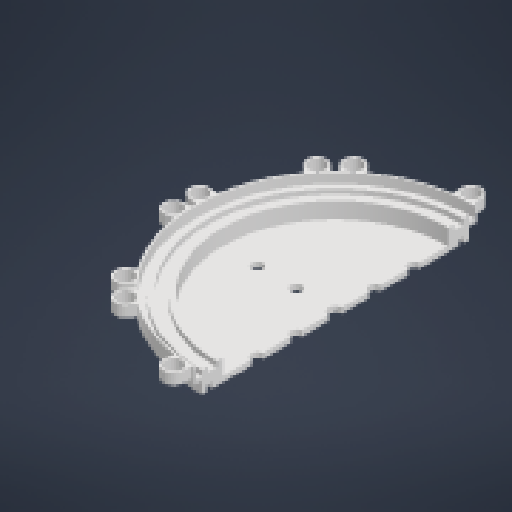
# Autodesk Inventor part: base frame
Saved by Autodesk Inventor 2026 (Build 300175050, 175E)
## iProperties
Created: 2026-03-26
Part Number: base frame
Material: Generic
Document SubType Name: Modeling
Designer: sniel
Density: 1 g/cm^3
Appearance: Default
Author: sniel
Autodesk Inventor part; units mm, degrees
ref_plane "YZ Plane" through (0, 0, 0) normal (1, 0, 0) x (0, 1, 0)
ref_plane "XZ Plane" through (0, 0, 0) normal (0, 1, 0) x (-1, 0, 0)
ref_plane "XY Plane" through (0, 0, 0) normal (0, 0, 1) x (1, 0, 0)
sketch "Sketch1" plane through (0, 0, 0) normal (0, 0, 1) x (1, 0, 0)
  line L0 (-117.014, 29.8572) -> (-117.014, 27.8572)
  line L1 (-119.014, 27.8572) -> (-119.014, 29.8572)
  line L2 (-0.014, 29.8572) -> (-125.014, 29.8572)
  line L3 (-0.014, 27.8572) -> (-119.014, 27.8572)
  line L4 (-113.014, 27.8572) -> (-113.014, 29.8572)
  line L5 (-111.014, 29.8572) -> (-111.014, 27.8572)
  line L6 (-105.014, 14.8572) -> (-105.014, 29.8572)
  line L7 (-0.014, 34.8572) -> (-130.014, 34.8572)
  line L8 (-100.014, 34.8572) -> (-100.014, 19.8572)
  line L9 (-130.014, 24.8572) -> (-130.014, 34.8572)
  line L10 (-0.014, 24.8572) -> (-130.014, 24.8572)
  line L11 (-0.014, 14.8572) -> (-105.014, 14.8572)
  line L12 (-100.014, 19.8572) -> (-0.014, 19.8572)
  line L13 (-125.014, 29.8572) -> (-125.014, 24.8572)
  line L14 (-125.014, 29.8572) -> (-124.814, 29.8572)
  line L15 (-124.814, 29.8572) -> (-124.814, 29.6572)
  line L16 (-124.814, 29.6572) -> (-125.014, 29.6572)
  line L17 (-125.014, 29.6572) -> (-125.014, 29.8572)
  line L18 (-119.014, 29.8572) -> (-119.214, 29.8572)
  line L19 (-119.214, 29.8572) -> (-119.214, 29.6572)
  line L20 (-119.214, 29.6572) -> (-119.014, 29.6572)
  line L21 (-119.014, 29.6572) -> (-119.014, 29.8572)
  line L22 (-111.014, 29.8572) -> (-110.814, 29.8572)
  line L23 (-110.814, 29.8572) -> (-110.814, 29.6572)
  line L24 (-110.814, 29.6572) -> (-111.014, 29.6572)
  line L25 (-111.014, 29.6572) -> (-111.014, 29.8572)
  line L26 (-105.014, 29.8572) -> (-105.214, 29.8572)
  line L27 (-105.214, 29.8572) -> (-105.214, 29.6572)
  line L28 (-105.214, 29.6572) -> (-105.014, 29.6572)
  line L29 (-105.014, 29.6572) -> (-105.014, 29.8572)
  line L30 (-124.814, 29.6572) -> (-119.214, 29.6572)
  line L31 (-119.214, 29.6572) -> (-119.214, 9.6572)
  line L32 (-119.214, 9.6572) -> (-124.814, 9.6572)
  line L33 (-124.814, 9.6572) -> (-124.814, 29.6572)
  line L34 (-110.814, 29.6572) -> (-105.214, 29.6572)
  line L35 (-105.214, 29.6572) -> (-105.214, 9.6572)
  line L36 (-105.214, 9.6572) -> (-110.814, 9.6572)
  line L37 (-110.814, 9.6572) -> (-110.814, 29.6572)
  line L38 (-119.014, 27.8572) -> (-117.014, 27.8572)
  line L39 (-117.014, 27.8572) -> (-117.014, 26.8572)
  line L40 (-117.014, 26.8572) -> (-119.014, 26.8572)
  line L41 (-119.014, 26.8572) -> (-119.014, 27.8572)
  line L42 (-113.014, 27.8572) -> (-111.014, 27.8572)
  line L43 (-111.014, 27.8572) -> (-111.014, 26.8572)
  line L44 (-111.014, 26.8572) -> (-113.014, 26.8572)
  line L45 (-113.014, 26.8572) -> (-113.014, 27.8572)
  line L46 (-119.214, 26.8572) -> (-110.814, 26.8572)
  line L47 (-110.814, 26.8572) -> (-110.814, 24.8572)
  line L48 (-110.814, 24.8572) -> (-119.214, 24.8572)
  line L49 (-119.214, 24.8572) -> (-119.214, 26.8572)
  line L50 (-124.814, 9.6572) -> (-0.014, 9.6572)
  line L51 (-0.014, 9.6572) -> (-0.014, 14.6572)
  line L52 (-0.014, 14.6572) -> (-124.814, 14.6572)
  line L53 (-124.814, 14.6572) -> (-124.814, 9.6572)
  line L54 (-124.814, 24.8572) -> (-125.014, 24.8572)
  line L55 (-125.014, 24.8572) -> (-125.014, 24.6572)
  line L56 (-125.014, 24.6572) -> (-124.814, 24.6572)
  line L57 (-124.814, 24.6572) -> (-124.814, 24.8572)
  line L58 (-124.814, 24.6572) -> (-132.014, 24.6572)
  line L59 (-132.014, 24.6572) -> (-132.014, 20.6572)
  line L60 (-132.014, 20.6572) -> (-124.814, 20.6572)
  line L61 (-124.814, 20.6572) -> (-124.814, 24.6572)
  line L62 (-132.014, 24.6572) -> (-130.214, 24.6572)
  line L63 (-130.214, 24.6572) -> (-130.214, 34.8572)
  line L64 (-130.214, 34.8572) -> (-132.014, 34.8572)
  line L65 (-132.014, 34.8572) -> (-132.014, 24.6572)
  line L66 (-0.014, 9.6572) -> (-6.014, 9.6572)
  line L67 (-6.014, 9.6572) -> (-6.014, 14.6572)
  line L68 (-6.014, 14.6572) -> (-0.014, 14.6572)
  line L69 (-0.014, 14.6572) -> (-0.014, 9.6572)
  line L70 (-119.014, 27.3572) -> (-117.014, 27.3572)
  line L71 (-117.014, 27.3572) -> (-117.014, 26.8572)
  line L72 (-117.014, 26.8572) -> (-119.014, 26.8572)
  line L73 (-119.014, 26.8572) -> (-119.014, 27.3572)
  line L74 (-113.014, 27.3572) -> (-111.014, 27.3572)
  line L75 (-111.014, 27.3572) -> (-111.014, 26.8572)
  line L76 (-111.014, 26.8572) -> (-113.014, 26.8572)
  line L77 (-113.014, 26.8572) -> (-113.014, 27.3572)
  line L78 (0, -6.9714) -> (0, 41.8287) projected
  line L79 (-115.014, 29.8572) -> (-115.014, 24.3572)
  line L80 (-110.814, 23.8572) -> (-119.214, 23.8572)
  line L81 (-110.814, 26.8572) -> (-113.014, 26.8572)
  line L82 (-113.014, 26.8572) -> (-113.014, 23.8572)
  line L83 (-113.014, 23.8572) -> (-110.814, 23.8572)
  line L84 (-110.814, 23.8572) -> (-110.814, 26.8572)
  line L85 (-117.014, 26.8572) -> (-119.214, 26.8572)
  line L86 (-119.214, 26.8572) -> (-119.214, 23.8572)
  line L87 (-119.214, 23.8572) -> (-117.014, 23.8572)
  line L88 (-117.014, 23.8572) -> (-117.014, 26.8572)
  line L89 (-110.814, 24.3572) -> (-119.214, 24.3572)
  point P0 (0, 0)
  point P1 (-105.214, 14.6572)
  point P2 (-113.014, 24.8572)
  point P3 (-115.014, 23.8572)
  point P4 (-115.014, 24.8572)
  point P5 (-117.014, 24.8572)
  dimension "d0" = 0.2
  dimension "d1" = 0.2
  dimension "d2" = 0.2
  dimension "d3" = 0.2
  dimension "d4" = 0.2
  dimension "d5" = 0.2
  dimension "d6" = 0.2
  dimension "d7" = 0.2
  dimension "d8" = 20
  dimension "d9" = 20
  dimension "d10" = 1
  dimension "d11" = 1
  dimension "d12" = 2
  dimension "d13" = 5
  dimension "d14" = 0.2
  dimension "d15" = 7.2
  dimension "d16" = 4
  dimension "d17" = 1.8
  dimension "d18" = 6
  dimension "d86" = 5.5
  constraints: 178 end point, 36 parallel, 20 perpendicular, 18 horizontal, 11 point on line, 2 midpoint, 1 vertical
  measures "d0" distance of L15.end L16.end
  measures "d1" distance of L14.end L15.end
  measures "d2" distance of L20.end L19.end
  measures "d3" distance of L19.end L18.end
  measures "d4" distance of L23.end L24.end
  measures "d5" distance of L22.end L23.end
  measures "d6" distance of L28.end L27.end
  measures "d7" distance of L27.end L26.end
  measures "d8" distance of L30.end L31.end
  measures "d9" distance of L34.end L35.end
  measures "d10" distance of L38.end L39.end
  measures "d11" distance of L42.end L43.end
  measures "d12" distance of L46.end L47.end
  measures "d13" distance of L51.end L50.end
  measures "d14" distance of L55.end L54.end
  measures "d15" distance of L60.end L59.end
  measures "d16" distance of L59.end L58.end
  measures "d17" distance of L64.end L63.end
  measures "d18" distance of L67.end L68.end
  measures "d86" distance of L79.start L79.end
revolve "Revolution1" add sketch "Sketch1" angle 360 about axis through (0, -10, 0) along (0, 1, 0) contours L31 L10 L33 L30 | L79 L89 L88 L10 | L10 L82 L89 L79 | L88 L89 L31 L10 | L37 L34 L35 L3 | L3 L35 L10 L37 | L10 L37 L89 L82 | L89 L82 L80 L88 | L31 L52 L33 L10 | L88 L80 L31 L89 | L10 L35 L52 L37 | L89 L37 L80 L82 | L80 L37 L52 L31 | L33 L60 L59 L58 L56 | L52 L67 L50 L35 | L35 L36 L37 L52 | L52 L37 L50 L31 | L31 L32 L33 L52 | L58 L65 L64 L63
sketch "Sketch3" plane through (0, 29.6572, 0) normal (0, 1, 0) x (1, 0, 0)
  circle A0 centre (0, 0) radius 132.014 projected
  circle A1 centre (0, 0) radius 6.014 projected
  line L0 (0, 0) -> (-93.348, -93.348)
  line L1 (0, 0) -> (132.014, 0) construction
  line L2 (0, 0) -> (0, -132.014)
  line L3 (0, 0) -> (-84.857, -101.1286)
  line L4 (0, 0) -> (160.5313, 0) construction
  line L5 (-84.857, -101.1286) -> (-94.4988, -112.6193)
  circle A2 centre (0, 0) radius 130.214 projected
  line L6 (0, 0) -> (-11.5058, -131.5116)
  line L7 (0, 0) -> (132.014, 0) construction
  line L8 (-11.5058, -131.5116) -> (-12.8131, -146.4546)
  circle A3 centre (-12.1594, -138.9831) radius 7.5
  circle A4 centre (-89.6779, -106.8739) radius 7.5
  circle A5 centre (-12.1594, -138.9831) radius 9.3
  circle A6 centre (-89.6779, -106.8739) radius 9.3
  circle A7 centre (0, 0) radius 139.514
  line L9 (-2.873, -139.4844) -> (0, 0)
  line L10 (-21.3919, -137.8642) -> (0, 0)
  line L11 (-82.3584, -112.6111) -> (0, 0)
  line L12 (-96.5989, -100.6619) -> (0, 0)
  point P0 (-91.4059, -95.2505)
  point P1 (-77.9309, -106.5573)
  point P2 (-2.7185, -131.986)
  point P3 (-20.2419, -130.4529)
  dimension "d22" = 135
  dimension "d23" = 130
  dimension "d24" = 15
  dimension "d25" = 95
  dimension "d26" = 15
  constraints: 26 end point, 13 point on circle, 3 centre point, 3 coincident, 3 horizontal, 2 equal length, 2 midpoint, 1 vertical, 6 other
  measures "d22" angle of L0 L1
  measures "d23" angle of L3 L4
  measures "d24" distance of L3.end L5.end
  measures "d25" angle of L6 L7
  measures "d26" distance of L6.end L8.end
extrude "Extrusion2" add sketch "Sketch3" along normal mid plane 10.4 contours A0 A6 L12 | L9 A5 A0 | A0 A4 A7 L12 A6 | A5 L9 A7 A3 A0 | A6 A0 L11 | A0 A6 A7 A4 | A7 A4 A6 | A3 A7 A5 A0 | A5 A7 A3 | A5 L10 A0
pattern_circular "Circular Pattern1" count 8 over 360 about axis through (0, -10, 0) along (0, 1, 0) of "Extrusion2"
sketch "Sketch5" plane through (0, 9.6572, 0) normal (0, -1, 0) x (1, 0, 0)
  circle A0 centre (0, 0) radius 132.014 projected
  arc A1 (-2.7185, -131.986) -> (2.7185, -131.986) centre (0, 0) ccw projected
  line L0 (0, -10) -> (26.9875, -10) construction
  line L1 (41.275, 0) -> (-30.9983, 0)
  line L2 (-7.5, -120.025) -> (7.5, -120.025)
  line L3 (7.5, -120.025) -> (7.5, -115.025)
  line L4 (7.5, -115.025) -> (-7.5, -115.025)
  line L5 (-7.5, -115.025) -> (-7.5, -120.025)
  line L6 (-7.5, -120.025) -> (7.5, -115.025) construction
  line L7 (7.5, -120.025) -> (-7.5, -115.025) construction
  line L8 (10, -122.525) -> (5, -122.525)
  line L9 (5, -122.525) -> (5, -112.525)
  line L10 (5, -112.525) -> (10, -112.525)
  line L11 (10, -112.525) -> (10, -122.525)
  line L12 (10, -122.525) -> (5, -112.525) construction
  line L13 (5, -122.525) -> (10, -112.525) construction
  line L14 (-5, -122.525) -> (-10, -122.525)
  line L15 (-10, -122.525) -> (-10, -112.525)
  line L16 (-10, -112.525) -> (-5, -112.525)
  line L17 (-5, -112.525) -> (-5, -122.525)
  line L18 (-5, -122.525) -> (-10, -112.525) construction
  line L19 (-10, -122.525) -> (-5, -112.525) construction
  line L20 (0, 0) -> (0, -115)
  line L21 (5, 112.525) -> (10, 112.525)
  line L22 (-10, 122.525) -> (-10, 112.525)
  line L23 (7.5, 115.025) -> (-7.5, 115.025)
  line L24 (-7.5, 115.025) -> (-7.5, 120.025)
  line L25 (-7.5, 120.025) -> (7.5, 120.025)
  line L26 (7.5, 120.025) -> (7.5, 115.025)
  line L27 (-7.5, 120.025) -> (7.5, 115.025) construction
  line L28 (7.5, 120.025) -> (-7.5, 115.025) construction
  line L29 (10, 122.525) -> (5, 122.525)
  line L30 (10, 112.525) -> (10, 122.525)
  line L31 (10, 122.525) -> (5, 112.525) construction
  line L32 (5, 122.525) -> (10, 112.525) construction
  line L33 (5, 122.525) -> (5, 112.525)
  line L34 (-5, 122.525) -> (-10, 122.525)
  line L35 (-5, 112.525) -> (-5, 122.525)
  line L36 (-5, 122.525) -> (-10, 112.525) construction
  line L37 (-10, 122.525) -> (-5, 112.525) construction
  line L38 (-10, 112.525) -> (-5, 112.525)
  line L39 (0, 0) -> (0, 115)
  arc A2 (131.986, -2.7185) -> (131.986, 2.7185) centre (0, 0) ccw
  line L40 (10, 0) -> (10, 26.9875) construction
  line L41 (0, 41.275) -> (0, -30.9983)
  line L42 (112.525, 5) -> (112.525, 10)
  line L43 (122.525, -10) -> (112.525, -10)
  line L44 (115.025, 7.5) -> (115.025, -7.5)
  line L45 (115.025, -7.5) -> (120.025, -7.5)
  line L46 (120.025, -7.5) -> (120.025, 7.5)
  line L47 (120.025, 7.5) -> (115.025, 7.5)
  line L48 (120.025, -7.5) -> (115.025, 7.5) construction
  line L49 (120.025, 7.5) -> (115.025, -7.5) construction
  line L50 (122.525, 10) -> (122.525, 5)
  line L51 (112.525, 10) -> (122.525, 10)
  line L52 (122.525, 10) -> (112.525, 5) construction
  line L53 (122.525, 5) -> (112.525, 10) construction
  line L54 (122.525, 5) -> (112.525, 5)
  line L55 (122.525, -5) -> (122.525, -10)
  line L56 (112.525, -5) -> (122.525, -5)
  line L57 (122.525, -5) -> (112.525, -10) construction
  line L58 (122.525, -10) -> (112.525, -5) construction
  line L59 (112.525, -10) -> (112.525, -5)
  line L60 (0, 0) -> (115, 0)
  line L61 (-122.525, 5) -> (-112.525, 5)
  line L62 (-120.025, 7.5) -> (-115.025, 7.5)
  line L63 (-120.025, -7.5) -> (-115.025, 7.5) construction
  line L64 (-120.025, 7.5) -> (-115.025, -7.5) construction
  line L65 (-112.525, 5) -> (-112.525, 10)
  line L66 (-112.525, 10) -> (-122.525, 10)
  line L67 (-122.525, 10) -> (-112.525, 5) construction
  line L68 (-122.525, 5) -> (-112.525, 10) construction
  line L69 (-120.025, -7.5) -> (-120.025, 7.5)
  line L70 (-122.525, 10) -> (-122.525, 5)
  line L71 (0, 0) -> (-115, 0)
  line L72 (-115.025, 7.5) -> (-115.025, -7.5)
  line L73 (-115.025, -7.5) -> (-120.025, -7.5)
  line L74 (-112.525, -5) -> (-122.525, -5)
  line L75 (-122.525, -5) -> (-122.525, -10)
  line L76 (-122.525, -10) -> (-112.525, -5) construction
  line L77 (-112.525, -10) -> (-112.525, -5)
  line L78 (-122.525, -5) -> (-112.525, -10) construction
  line L79 (-122.525, -10) -> (-112.525, -10)
  point P0 (7.5, -117.525)
  point P1 (-7.5, -117.525)
  point P2 (-5, -120.025)
  point P3 (5, -120.025)
  point P4 (5, -115.025)
  point P5 (-5, -115.025)
  point P6 (-7.5, 117.525)
  point P7 (7.5, 117.525)
  point P8 (-5, 115.025)
  point P9 (5, 115.025)
  point P10 (5, 120.025)
  point P11 (-5, 120.025)
  point P12 (0, 0)
  point P13 (0, 0)
  point P14 (117.525, -7.5)
  point P15 (117.525, 7.5)
  point P16 (-117.525, 7.5)
  point P17 (-117.525, -7.5)
  point P18 (120.025, -5)
  point P19 (120.025, 5)
  point P20 (115.025, 5)
  point P21 (115.025, -5)
  point P22 (-120.025, 5)
  point P23 (-120.025, -5)
  point P24 (-115.025, -5)
  point P25 (-115.025, 5)
  dimension "d62" = 115
  dimension "d89" = 115
  constraints: 160 end point, 30 symmetric about line, 2 horizontal, 2 perpendicular, 2 point on circle, 1 centre point
  measures "d62" distance of L20.start L20.end
  measures "d89" distance of L60.start L60.end
extrude "Extrusion4" cut sketch "Sketch5" against normal blind 5 contours L5 L4 L17 L2 | L2 L17 L14 L15 L16 L4 L5 | L17 L4 L9 L2 | L9 L4 L3 L2 | L2 L3 L4 L9 L10 L11 L8 | L33 L23 L26 L25 L29 L30 L21 | L33 L25 L26 L23 | L23 L35 L25 L33 | L35 L38 L22 L34 L25 L24 L23 | L23 L24 L25 L35 | L42 L51 L50 L54 L46 L47 L44 | L54 L46 L56 L44 | L44 L47 L46 L54 | L56 L46 L45 L44 | L44 L45 L46 L56 L55 L43 L59 | L70 L66 L65 L61 L72 L62 L69 | L69 L62 L72 L61 | L61 L72 L74 L69 | L74 L72 L73 L69 | L69 L73 L72 L74 L77 L79 L75
sketch "Sketch6" plane through (0, 9.6572, 0) normal (0, -1, 0) x (1, 0, 0)
  arc A0 (-5.3566, 19.1544) -> (-6.464, 18.848) centre (-0.6442, -0.0297) ccw projected
  arc A1 (-3.9705, 16.9967) -> (-5.3566, 19.1544) centre (-15.5742, 11.0669) ccw projected
  arc A2 (-3.9236, 16.861) -> (-3.9705, 16.9967) centre (-22.8251, 10.402) ccw projected
  arc A3 (-3.9028, 16.8624) -> (-3.9236, 16.861) centre (2.0614, -72.6393) ccw projected
  arc A4 (-3.6762, 16.3816) -> (-3.9028, 16.8624) centre (-15.5742, 11.0669) ccw projected
  arc A5 (-2.7169, 16.5302) -> (-3.6762, 16.3816) centre (-0.6442, -0.0297) ccw projected
  arc A6 (-1.9537, 19.6813) -> (-2.7169, 16.5302) centre (10.2313, 15.0621) ccw projected
  arc A7 (-0.8054, 19.724) -> (-1.9537, 19.6813) centre (-0.6442, -0.0297) ccw projected
  arc A8 (0.1902, 16.6385) -> (-0.8054, 19.724) centre (-12.6127, 14.2109) ccw projected
  arc A9 (1.158, 16.5618) -> (0.1902, 16.6385) centre (-0.6442, -0.0297) ccw projected
  arc A10 (1.3482, 17.0581) -> (1.158, 16.5618) centre (13.4185, 12.1472) ccw projected
  arc A11 (1.369, 17.0582) -> (1.3482, 17.0581) centre (2.0614, -72.6393) ccw projected
  arc A12 (1.4057, 17.197) -> (1.369, 17.0582) centre (20.6987, 12.0238) ccw projected
  arc A13 (2.6273, 19.4519) -> (1.4057, 17.197) centre (13.4185, 12.1472) ccw projected
  arc A14 (3.7545, 19.2287) -> (2.6273, 19.4519) centre (-0.6442, -0.0297) ccw projected
  arc A15 (4.0117, 15.9968) -> (3.7545, 19.2287) centre (-9.006, 16.5872) ccw projected
  arc A16 (4.9357, 15.6989) -> (4.0117, 15.9968) centre (-0.6442, -0.0297) ccw projected
  arc A17 (7.0319, 18.1723) -> (4.9357, 15.6989) centre (15.8477, 8.5759) ccw projected
  arc A18 (8.0773, 17.6952) -> (7.0319, 18.1723) centre (-0.6442, -0.0297) ccw projected
  arc A19 (7.5821, 14.491) -> (8.0773, 17.6952) centre (-4.9485, 18.0676) ccw projected
  arc A20 (8.4125, 13.9881) -> (7.5821, 14.491) centre (-0.6442, -0.0297) ccw projected
  arc A21 (11.0227, 15.9114) -> (8.4125, 13.9881) centre (17.3877, 4.5407) ccw projected
  arc A22 (11.9298, 15.2061) -> (11.0227, 15.9114) centre (-0.6442, -0.0297) ccw projected
  arc A23 (10.7091, 12.2025) -> (11.9298, 15.2061) centre (-0.6589, 18.5724) ccw projected
  arc A24 (11.4012, 11.5216) -> (10.7091, 12.2025) centre (-0.6442, -0.0297) ccw projected
  arc A25 (14.3845, 12.7912) -> (11.4012, 11.5216) centre (17.9557, 0.259) ccw projected
  arc A26 (15.1045, 11.8956) -> (14.3845, 12.7912) centre (-0.6442, -0.0297) ccw projected
  arc A27 (13.224, 9.2545) -> (15.1045, 11.8956) centre (3.6314, 18.0744) ccw projected
  arc A28 (13.7404, 8.4324) -> (13.224, 9.2545) centre (-0.6442, -0.0297) ccw projected
  arc A29 (16.9361, 8.9797) -> (13.7404, 8.4324) centre (17.5209, -4.0382) ccw projected
  arc A30 (17.4302, 7.9423) -> (16.9361, 8.9797) centre (-0.6442, -0.0297) ccw projected
  arc A31 (14.9913, 5.806) -> (17.4302, 7.9423) centre (7.6912, 16.6004) ccw projected
  arc A32 (15.3042, 4.887) -> (14.9913, 5.806) centre (-0.6442, -0.0297) ccw projected
  arc A33 (18.5399, 4.6826) -> (15.3042, 4.887) centre (16.1068, -8.1193) ccw projected
  arc A34 (18.7815, 3.5591) -> (18.5399, 4.6826) centre (-0.6442, -0.0297) ccw projected
  arc A35 (15.9157, 2.0429) -> (18.7815, 3.5591) centre (11.3017, 14.2298) ccw projected
  arc A36 (16.0081, 1.0765) -> (15.9157, 2.0429) centre (-0.6442, -0.0297) ccw projected
  arc A37 (19.1095, 0.1314) -> (16.0081, 1.0765) centre (13.7897, -11.7644) ccw projected
  arc A38 (19.0855, -1.0175) -> (19.1095, 0.1314) centre (-0.6442, -0.0297) ccw projected
  arc A39 (15.9473, -1.832) -> (19.0855, -1.0175) centre (14.2682, 11.0905) ccw projected
  arc A40 (15.8144, -2.7936) -> (15.9473, -1.832) centre (-0.6442, -0.0297) ccw projected
  arc A41 (18.6142, -4.4285) -> (15.8144, -2.7936) centre (10.6945, -14.7767) ccw projected
  arc A42 (18.3259, -5.5408) -> (18.6142, -4.4285) centre (-0.6442, -0.0297) ccw projected
  arc A43 (15.0844, -5.6096) -> (18.3259, -5.5408) centre (16.4307, 7.3517) ccw projected
  arc A44 (14.7334, -6.5147) -> (15.0844, -5.6096) centre (-0.6442, -0.0297) ccw projected
  arc A45 (17.0807, -8.7512) -> (14.7334, -6.5147) centre (6.9879, -16.9941) ccw projected
  arc A46 (16.5436, -9.7671) -> (17.0807, -8.7512) centre (-0.6442, -0.0297) ccw projected
  arc A47 (13.3736, -9.0865) -> (16.5436, -9.7671) centre (17.6728, 3.215) ccw projected
  arc A48 (12.8233, -9.8863) -> (13.3736, -9.0865) centre (-0.6442, -0.0297) ccw projected
  arc A49 (14.5916, -12.6038) -> (12.8233, -9.8863) centre (2.8699, -18.2969) ccw projected
  arc A50 (13.8347, -13.4684) -> (14.5916, -12.6038) centre (-0.6442, -0.0297) ccw projected
  arc A51 (10.9071, -12.0751) -> (13.8347, -13.4684) centre (17.9273, -1.0967) ccw projected
  arc A52 (10.1872, -12.7264) -> (10.9071, -12.0751) centre (-0.6442, -0.0297) ccw projected
  arc A53 (11.2811, -15.7785) -> (10.1872, -12.7264) centre (-1.4375, -18.615) ccw projected
  arc A54 (10.3453, -16.4452) -> (11.2811, -15.7785) centre (-0.6442, -0.0297) ccw projected
  arc A55 (7.8179, -14.4144) -> (10.3453, -16.4452) centre (17.1806, -5.3508) ccw projected
  arc A56 (6.9672, -14.8821) -> (7.8179, -14.4144) centre (-0.6442, -0.0297) ccw projected
  arc A57 (7.3278, -18.1042) -> (6.9672, -14.8821) centre (-5.7022, -17.9311) ccw projected
  arc A58 (6.2634, -18.5371) -> (7.3278, -18.1042) centre (-0.6442, -0.0297) ccw projected
  arc A59 (4.2725, -15.9781) -> (6.2634, -18.5371) centre (15.4731, -9.3181) ccw projected
  arc A60 (3.3369, -16.237) -> (4.2725, -15.9781) centre (-0.6442, -0.0297) ccw projected
  arc A61 (2.9446, -19.4554) -> (3.3369, -16.237) centre (-9.6942, -16.2821) ccw projected
  arc A62 (1.8091, -19.6312) -> (2.9446, -19.4554) centre (-0.6442, -0.0297) ccw projected
  arc A63 (0.462, -16.6821) -> (1.8091, -19.6312) centre (12.8966, -12.7846) ccw projected
  arc A64 (-0.5081, -16.7183) -> (0.462, -16.6821) centre (-0.6442, -0.0297) ccw projected
  arc A65 (-1.632, -19.7595) -> (-0.5081, -16.7183) centre (-13.1983, -13.757) ccw projected
  arc A66 (-2.7775, -19.6687) -> (-1.632, -19.7595) centre (-0.6442, -0.0297) ccw projected
  arc A67 (-3.4081, -16.4884) -> (-2.7775, -19.6687) centre (9.5901, -15.5635) ccw projected
  arc A68 (-4.3604, -16.2998) -> (-3.4081, -16.4884) centre (-0.6442, -0.0297) ccw projected
  arc A69 (-6.1553, -18.9999) -> (-4.3604, -16.2998) centre (-16.0256, -10.4918) ccw projected
  arc A70 (-7.249, -18.6473) -> (-6.1553, -18.9999) centre (-0.6442, -0.0297) ccw projected
  arc A71 (-7.1292, -15.4073) -> (-7.249, -18.6473) centre (5.7319, -17.505) ccw projected
  arc A72 (-8.0124, -15.0042) -> (-7.1292, -15.4073) centre (-0.6442, -0.0297) ccw projected
  arc A73 (-10.3816, -17.2176) -> (-8.0124, -15.0042) centre (-18.0237, -6.6626) ccw projected
  arc A74 (-11.3645, -16.6223) -> (-10.3816, -17.2176) centre (-0.6442, -0.0297) ccw projected
  arc A75 (-10.5008, -13.4973) -> (-11.3645, -16.6223) centre (1.5299, -18.5044) ccw projected
  arc A76 (-11.2672, -12.9014) -> (-10.5008, -13.4973) centre (-0.6442, -0.0297) ccw projected
  arc A77 (-14.0829, -14.5087) -> (-11.2672, -12.9014) centre (-19.0849, -2.4758) ccw projected
  arc A78 (-14.9021, -13.7028) -> (-14.0829, -14.5087) centre (-0.6442, -0.0297) ccw projected
  arc A79 (-13.3409, -10.8612) -> (-14.9021, -13.7028) centre (-2.7892, -18.5078) ccw projected
  arc A80 (-13.9492, -10.1046) -> (-13.3409, -10.8612) centre (-0.6442, -0.0297) ccw projected
  arc A81 (-17.0597, -11.0192) -> (-13.9492, -10.1046) centre (-19.1519, 1.8428) ccw projected
  arc A82 (-17.671, -10.0462) -> (-17.0597, -11.0192) centre (-0.6442, -0.0297) ccw projected
  arc A83 (-15.4966, -7.6412) -> (-17.671, -10.0462) centre (-6.9927, -17.5151) ccw projected
  arc A84 (-15.914, -6.7647) -> (-15.4966, -7.6412) centre (-0.6442, -0.0297) ccw projected
  arc A85 (-19.1516, -6.9373) -> (-15.914, -6.7647) centre (-18.2212, 6.0605) ccw projected
  arc A86 (-19.5219, -5.8495) -> (-19.1516, -6.9373) centre (-0.6442, -0.0297) ccw projected
  arc A87 (-16.8515, -4.0108) -> (-19.5219, -5.8495) centre (-10.854, -15.5797) ccw projected
  arc A88 (-17.0556, -3.0617) -> (-16.8515, -4.0108) centre (-0.6442, -0.0297) ccw projected
  arc A89 (-20.2457, -2.483) -> (-17.0556, -3.0617) centre (-16.3429, 9.9499) ccw projected
  arc A90 (-20.3552, -1.3392) -> (-20.2457, -2.483) centre (-0.6442, -0.0297) ccw projected
  arc A91 (-17.3328, -0.1659) -> (-20.3552, -1.3392) centre (-14.1649, -12.806) ccw projected
  arc A92 (-17.3125, 0.8047) -> (-17.3328, -0.1659) centre (-0.6442, -0.0297) ccw projected
  arc A93 (-20.2832, 2.1035) -> (-17.3125, 0.8047) centre (-13.6183, 13.3012) ccw projected
  arc A94 (-20.1259, 3.2418) -> (-20.2832, 2.1035) centre (-0.6442, -0.0297) ccw projected
  arc A95 (-16.9143, 3.6865) -> (-20.1259, 3.2418) centre (-16.7468, -9.3435) ccw projected
  arc A96 (-16.6707, 4.6262) -> (-16.9143, 3.6865) centre (-0.6442, -0.0297) ccw projected
  arc A97 (-19.2618, 6.5751) -> (-16.6707, 4.6262) centre (-10.1942, 15.9339) ccw projected
  arc A98 (-18.8463, 7.6464) -> (-19.2618, 6.5751) centre (-0.6442, -0.0297) ccw projected
  arc A99 (-15.6188, 7.3384) -> (-18.8463, 7.6464) centre (-18.4607, -5.379) ccw projected
  arc A100 (-15.165, 8.1967) -> (-15.6188, 7.3384) centre (-0.6442, -0.0297) ccw projected
  arc A101 (-17.2368, 10.6905) -> (-15.165, 8.1967) centre (-6.2554, 17.706) ccw projected
  arc A102 (-16.5854, 11.6372) -> (-17.2368, 10.6905) centre (-0.6442, -0.0297) ccw projected
  arc A103 (-13.5159, 10.5932) -> (-16.5854, 11.6372) centre (-19.2141, -1.126) ccw projected
  arc A104 (-12.8765, 11.3236) -> (-13.5159, 10.5932) centre (-0.6442, -0.0297) ccw projected
  arc A105 (-14.3173, 14.2281) -> (-12.8765, 11.3236) centre (-2.014, 18.5219) ccw projected
  arc A106 (-13.4652, 14.999) -> (-14.3173, 14.2281) centre (-0.6442, -0.0297) ccw projected
  arc A107 (-10.7191, 13.2752) -> (-13.4652, 14.999) centre (-18.9663, 3.186) ccw projected
  arc A108 (-9.9285, 13.8385) -> (-10.7191, 13.2752) centre (-0.6442, -0.0297) ccw projected
  arc A109 (-10.6607, 16.997) -> (-9.9285, 13.8385) centre (2.3013, 18.3378) ccw projected
  arc A110 (-9.6537, 17.5506) -> (-10.6607, 16.997) centre (-0.6442, -0.0297) ccw projected
  arc A111 (-7.3792, 15.24) -> (-9.6537, 17.5506) centre (-17.7309, 7.3247) ccw projected
  arc A112 (-6.48, 15.6058) -> (-7.3792, 15.24) centre (-0.6442, -0.0297) ccw projected
  arc A113 (-6.464, 18.848) -> (-6.48, 15.6058) centre (6.4577, 17.1634) ccw projected
  circle A114 centre (0, 0) radius 5 projected
  arc A115 (-6.6761, 89.6063) -> (-8.0622, 91.764) centre (-18.2798, 83.6765) ccw
  arc A116 (-8.0622, 91.764) -> (-9.1696, 91.4576) centre (-3.3498, 72.5799) ccw
  arc A117 (-9.1696, 91.4576) -> (-9.1856, 88.2154) centre (3.7521, 89.773) ccw
  arc A118 (-9.1856, 88.2154) -> (-10.0848, 87.8496) centre (-3.3498, 72.5799) ccw
  arc A119 (-10.0848, 87.8496) -> (-12.3593, 90.1602) centre (-20.4365, 79.9343) ccw
  arc A120 (-12.3593, 90.1602) -> (-13.3663, 89.6066) centre (-3.3498, 72.5799) ccw
  arc A121 (-13.3663, 89.6066) -> (-12.6341, 86.4481) centre (-0.4043, 90.9474) ccw
  arc A122 (-12.6341, 86.4481) -> (-13.4247, 85.8849) centre (-3.3498, 72.5799) ccw
  arc A123 (-13.4247, 85.8849) -> (-16.1708, 87.6086) centre (-21.6719, 75.7956) ccw
  arc A124 (-16.1708, 87.6086) -> (-17.0229, 86.8377) centre (-3.3498, 72.5799) ccw
  arc A125 (-17.0229, 86.8377) -> (-15.5821, 83.9332) centre (-4.7196, 91.1315) ccw
  arc A126 (-15.5821, 83.9332) -> (-16.2215, 83.2028) centre (-3.3498, 72.5799) ccw
  arc A127 (-16.2215, 83.2028) -> (-19.291, 84.2468) centre (-21.9197, 71.4836) ccw
  arc A128 (-19.291, 84.2468) -> (-19.9424, 83.3001) centre (-3.3498, 72.5799) ccw
  arc A129 (-19.9424, 83.3001) -> (-17.8706, 80.8063) centre (-8.961, 90.3156) ccw
  arc A130 (-17.8706, 80.8063) -> (-18.3244, 79.948) centre (-3.3498, 72.5799) ccw
  arc A131 (-18.3244, 79.948) -> (-21.5519, 80.256) centre (-21.1663, 67.2306) ccw
  arc A132 (-21.5519, 80.256) -> (-21.9674, 79.1847) centre (-3.3498, 72.5799) ccw
  arc A133 (-21.9674, 79.1847) -> (-19.3763, 77.2358) centre (-12.8999, 88.5435) ccw
  arc A134 (-19.3763, 77.2358) -> (-19.6199, 76.2961) centre (-3.3498, 72.5799) ccw
  arc A135 (-19.6199, 76.2961) -> (-22.8315, 75.8514) centre (-19.4524, 63.2661) ccw
  arc A136 (-22.8315, 75.8514) -> (-22.9888, 74.7131) centre (-3.3498, 72.5799) ccw
  arc A137 (-22.9888, 74.7131) -> (-20.0181, 73.4143) centre (-16.3239, 85.9108) ccw
  arc A138 (-20.0181, 73.4143) -> (-20.0384, 72.4438) centre (-3.3498, 72.5799) ccw
  arc A139 (-20.0384, 72.4438) -> (-23.0608, 71.2704) centre (-16.8705, 59.8036) ccw
  arc A140 (-23.0608, 71.2704) -> (-22.9514, 70.1266) centre (-3.3498, 72.5799) ccw
  arc A141 (-22.9514, 70.1266) -> (-19.7612, 69.5479) centre (-19.0485, 82.5595) ccw
  arc A142 (-19.7612, 69.5479) -> (-19.5571, 68.5988) centre (-3.3498, 72.5799) ccw
  arc A143 (-19.5571, 68.5988) -> (-22.2275, 66.7601) centre (-13.5596, 57.0299) ccw
  arc A144 (-22.2275, 66.7601) -> (-21.8572, 65.6723) centre (-3.3498, 72.5799) ccw
  arc A145 (-21.8572, 65.6723) -> (-18.6196, 65.8449) centre (-20.9268, 78.6701) ccw
  arc A146 (-18.6196, 65.8449) -> (-18.2022, 64.9684) centre (-3.3498, 72.5799) ccw
  arc A147 (-18.2022, 64.9684) -> (-20.3766, 62.5634) centre (-9.6983, 55.0945) ccw
  arc A148 (-20.3766, 62.5634) -> (-19.7653, 61.5904) centre (-3.3498, 72.5799) ccw
  arc A149 (-19.7653, 61.5904) -> (-16.6548, 62.505) centre (-21.8575, 74.4524) ccw
  arc A150 (-16.6548, 62.505) -> (-16.0465, 61.7484) centre (-3.3498, 72.5799) ccw
  arc A151 (-16.0465, 61.7484) -> (-17.6077, 58.9068) centre (-5.4948, 54.1018) ccw
  arc A152 (-17.6077, 58.9068) -> (-16.7885, 58.1009) centre (-3.3498, 72.5799) ccw
  arc A153 (-16.7885, 58.1009) -> (-13.9728, 59.7082) centre (-21.7905, 70.1338) ccw
  arc A154 (-13.9728, 59.7082) -> (-13.2064, 59.1123) centre (-3.3498, 72.5799) ccw
  arc A155 (-13.2064, 59.1123) -> (-14.0701, 55.9873) centre (-1.1757, 54.1052) ccw
  arc A156 (-14.0701, 55.9873) -> (-13.0872, 55.392) centre (-3.3498, 72.5799) ccw
  arc A157 (-13.0872, 55.392) -> (-10.718, 57.6054) centre (-20.7293, 65.947) ccw
  arc A158 (-10.718, 57.6054) -> (-9.8348, 57.2023) centre (-3.3498, 72.5799) ccw
  arc A159 (-9.8348, 57.2023) -> (-9.9546, 53.9623) centre (3.0263, 55.1046) ccw
  arc A160 (-9.9546, 53.9623) -> (-8.8609, 53.6098) centre (-3.3498, 72.5799) ccw
  arc A161 (-8.8609, 53.6098) -> (-7.066, 56.3098) centre (-18.7312, 62.1178) ccw
  arc A162 (-7.066, 56.3098) -> (-6.1137, 56.1212) centre (-3.3498, 72.5799) ccw
  arc A163 (-6.1137, 56.1212) -> (-5.4831, 52.941) centre (6.8845, 57.0461) ccw
  arc A164 (-5.4831, 52.941) -> (-4.3376, 52.8501) centre (-3.3498, 72.5799) ccw
  arc A165 (-4.3376, 52.8501) -> (-3.2137, 55.8913) centre (-15.9039, 58.8526) ccw
  arc A166 (-3.2137, 55.8913) -> (-2.2436, 55.9275) centre (-3.3498, 72.5799) ccw
  arc A167 (-2.2436, 55.9275) -> (-0.8965, 52.9784) centre (10.191, 59.825) ccw
  arc A168 (-0.8965, 52.9784) -> (0.239, 53.1542) centre (-3.3498, 72.5799) ccw
  arc A169 (0.239, 53.1542) -> (0.6312, 56.3726) centre (-12.3998, 56.3275) ccw
  arc A170 (0.6312, 56.3726) -> (1.5669, 56.6315) centre (-3.3498, 72.5799) ccw
  arc A171 (1.5669, 56.6315) -> (3.5578, 54.0725) centre (12.7675, 63.2915) ccw
  arc A172 (3.5578, 54.0725) -> (4.6222, 54.5055) centre (-3.3498, 72.5799) ccw
  arc A173 (4.6222, 54.5055) -> (4.2616, 57.7275) centre (-8.4078, 54.6785) ccw
  arc A174 (4.2616, 57.7275) -> (5.1123, 58.1952) centre (-3.3498, 72.5799) ccw
  arc A175 (5.1123, 58.1952) -> (7.6397, 56.1644) centre (14.475, 67.2588) ccw
  arc A176 (7.6397, 56.1644) -> (8.5755, 56.8311) centre (-3.3498, 72.5799) ccw
  arc A177 (8.5755, 56.8311) -> (7.4816, 59.8832) centre (-4.1431, 53.9946) ccw
  arc A178 (7.4816, 59.8832) -> (8.2015, 60.5345) centre (-3.3498, 72.5799) ccw
  arc A179 (8.2015, 60.5345) -> (11.1291, 59.1412) centre (15.2217, 71.5129) ccw
  arc A180 (11.1291, 59.1412) -> (11.886, 60.0058) centre (-3.3498, 72.5799) ccw
  arc A181 (11.886, 60.0058) -> (10.1177, 62.7234) centre (0.1643, 54.3127) ccw
  arc A182 (10.1177, 62.7234) -> (10.668, 63.5231) centre (-3.3498, 72.5799) ccw
  arc A183 (10.668, 63.5231) -> (13.838, 62.8425) centre (14.9672, 75.8246) ccw
  arc A184 (13.838, 62.8425) -> (14.3751, 63.8584) centre (-3.3498, 72.5799) ccw
  arc A185 (14.3751, 63.8584) -> (12.0278, 66.0949) centre (4.2823, 55.6155) ccw
  arc A186 (12.0278, 66.0949) -> (12.3788, 67) centre (-3.3498, 72.5799) ccw
  arc A187 (12.3788, 67) -> (15.6203, 67.0688) centre (13.7251, 79.9613) ccw
  arc A188 (15.6203, 67.0688) -> (15.9086, 68.1811) centre (-3.3498, 72.5799) ccw
  arc A189 (15.9086, 68.1811) -> (13.1088, 69.816) centre (7.9889, 57.8329) ccw
  arc A190 (13.1088, 69.816) -> (13.2417, 70.7777) centre (-3.3498, 72.5799) ccw
  arc A191 (13.2417, 70.7777) -> (16.3799, 71.5921) centre (11.5626, 83.7001) ccw
  arc A192 (16.3799, 71.5921) -> (16.4039, 72.741) centre (-3.3498, 72.5799) ccw
  arc A193 (16.4039, 72.741) -> (13.3025, 73.6861) centre (11.0841, 60.8453) ccw
  arc A194 (13.3025, 73.6861) -> (13.2101, 74.6525) centre (-3.3498, 72.5799) ccw
  arc A195 (13.2101, 74.6525) -> (16.0759, 76.1688) centre (8.5961, 86.8394) ccw
  arc A196 (16.0759, 76.1688) -> (15.8343, 77.2922) centre (-3.3498, 72.5799) ccw
  arc A197 (15.8343, 77.2922) -> (12.5986, 77.4966) centre (13.4012, 64.4903) ccw
  arc A198 (12.5986, 77.4966) -> (12.2857, 78.4156) centre (-3.3498, 72.5799) ccw
  arc A199 (12.2857, 78.4156) -> (14.7246, 80.5519) centre (4.9856, 89.21) ccw
  arc A200 (14.7246, 80.5519) -> (14.2305, 81.5893) centre (-3.3498, 72.5799) ccw
  arc A201 (14.2305, 81.5893) -> (11.0348, 81.042) centre (14.8153, 68.5714) ccw
  arc A202 (11.0348, 81.042) -> (10.5184, 81.8641) centre (-3.3498, 72.5799) ccw
  arc A203 (10.5184, 81.8641) -> (12.3989, 84.5053) centre (0.9258, 90.684) ccw
  arc A204 (12.3989, 84.5053) -> (11.6789, 85.4008) centre (-3.3498, 72.5799) ccw
  arc A205 (11.6789, 85.4008) -> (8.6955, 84.1313) centre (15.2501, 72.8686) ccw
  arc A206 (8.6955, 84.1313) -> (8.0035, 84.8121) centre (-3.3498, 72.5799) ccw
  arc A207 (8.0035, 84.8121) -> (9.2242, 87.8157) centre (-3.3646, 91.182) ccw
  arc A208 (9.2242, 87.8157) -> (8.3171, 88.5211) centre (-3.3498, 72.5799) ccw
  arc A209 (8.3171, 88.5211) -> (5.7069, 86.5977) centre (14.6821, 77.1503) ccw
  arc A210 (5.7069, 86.5977) -> (4.8765, 87.1006) centre (-3.3498, 72.5799) ccw
  arc A211 (4.8765, 87.1006) -> (5.3717, 90.3048) centre (-7.6541, 90.6772) ccw
  arc A212 (5.3717, 90.3048) -> (4.3263, 90.7819) centre (-3.3498, 72.5799) ccw
  arc A213 (4.3263, 90.7819) -> (2.2301, 88.3085) centre (13.1421, 81.1855) ccw
  arc A214 (2.2301, 88.3085) -> (1.3061, 88.6064) centre (-3.3498, 72.5799) ccw
  arc A215 (1.3061, 88.6064) -> (1.0489, 91.8383) centre (-11.7116, 89.1968) ccw
  arc A216 (1.0489, 91.8383) -> (-0.0783, 92.0615) centre (-3.3498, 72.5799) ccw
  arc A217 (-0.0783, 92.0615) -> (-1.2999, 89.8066) centre (10.7129, 84.7569) ccw
  arc A218 (-1.2999, 89.8066) -> (-1.3366, 89.6678) centre (17.9931, 84.6334) ccw
  arc A219 (-1.3366, 89.6678) -> (-1.3574, 89.6677) centre (-0.6442, -0.0297) ccw
  arc A220 (-1.3574, 89.6677) -> (-1.5476, 89.1714) centre (10.7129, 84.7569) ccw
  arc A221 (-1.5476, 89.1714) -> (-2.5154, 89.2481) centre (-3.3498, 72.5799) ccw
  arc A222 (-2.5154, 89.2481) -> (-3.511, 92.3337) centre (-15.3183, 86.8205) ccw
  arc A223 (-3.511, 92.3337) -> (-4.6593, 92.2909) centre (-3.3498, 72.5799) ccw
  arc A224 (-4.6593, 92.2909) -> (-5.4225, 89.1398) centre (7.5257, 87.6717) ccw
  arc A225 (-5.4225, 89.1398) -> (-6.3818, 88.9912) centre (-3.3498, 72.5799) ccw
  arc A226 (-6.3818, 88.9912) -> (-6.6085, 89.472) centre (-18.2798, 83.6765) ccw
  arc A227 (-6.6085, 89.472) -> (-6.6292, 89.4706) centre (-0.6442, -0.0297) ccw
  arc A228 (-6.6292, 89.4706) -> (-6.6761, 89.6063) centre (-25.5307, 83.0116) ccw
  circle A229 centre (-3.3498, 72.5799) radius 5
  arc A230 (-3.3263, 53.5389) -> (-4.7123, 55.6967) centre (-14.93, 47.6091) ccw
  arc A231 (-4.7123, 55.6967) -> (-5.8198, 55.3902) centre (0, 36.5125) ccw
  arc A232 (-5.8198, 55.3902) -> (-5.8357, 52.148) centre (7.1019, 53.7056) ccw
  arc A233 (-5.8357, 52.148) -> (-6.735, 51.7823) centre (0, 36.5125) ccw
  arc A234 (-6.735, 51.7823) -> (-9.0095, 54.0928) centre (-17.0866, 43.8669) ccw
  arc A235 (-9.0095, 54.0928) -> (-10.0164, 53.5392) centre (0, 36.5125) ccw
  arc A236 (-10.0164, 53.5392) -> (-9.2842, 50.3808) centre (2.9455, 54.88) ccw
  arc A237 (-9.2842, 50.3808) -> (-10.0749, 49.8175) centre (0, 36.5125) ccw
  arc A238 (-10.0749, 49.8175) -> (-12.8209, 51.5412) centre (-18.3221, 39.7282) ccw
  arc A239 (-12.8209, 51.5412) -> (-13.6731, 50.7703) centre (0, 36.5125) ccw
  arc A240 (-13.6731, 50.7703) -> (-12.2322, 47.8659) centre (-1.3697, 55.0642) ccw
  arc A241 (-12.2322, 47.8659) -> (-12.8717, 47.1354) centre (0, 36.5125) ccw
  arc A242 (-12.8717, 47.1354) -> (-15.9412, 48.1794) centre (-18.5698, 35.4162) ccw
  arc A243 (-15.9412, 48.1794) -> (-16.5926, 47.2328) centre (0, 36.5125) ccw
  arc A244 (-16.5926, 47.2328) -> (-14.5208, 44.7389) centre (-5.6111, 54.2482) ccw
  arc A245 (-14.5208, 44.7389) -> (-14.9745, 43.8807) centre (0, 36.5125) ccw
  arc A246 (-14.9745, 43.8807) -> (-18.2021, 44.1886) centre (-17.8165, 31.1633) ccw
  arc A247 (-18.2021, 44.1886) -> (-18.6176, 43.1173) centre (0, 36.5125) ccw
  arc A248 (-18.6176, 43.1173) -> (-16.0265, 41.1684) centre (-9.55, 52.4761) ccw
  arc A249 (-16.0265, 41.1684) -> (-16.2701, 40.2287) centre (0, 36.5125) ccw
  arc A250 (-16.2701, 40.2287) -> (-19.4817, 39.784) centre (-16.1026, 27.1987) ccw
  arc A251 (-19.4817, 39.784) -> (-19.6389, 38.6457) centre (0, 36.5125) ccw
  arc A252 (-19.6389, 38.6457) -> (-16.6682, 37.347) centre (-12.9741, 49.8435) ccw
  arc A253 (-16.6682, 37.347) -> (-16.6885, 36.3764) centre (0, 36.5125) ccw
  arc A254 (-16.6885, 36.3764) -> (-19.711, 35.2031) centre (-13.5206, 23.7362) ccw
  arc A255 (-19.711, 35.2031) -> (-19.6015, 34.0592) centre (0, 36.5125) ccw
  arc A256 (-19.6015, 34.0592) -> (-16.4114, 33.4805) centre (-15.6987, 46.4921) ccw
  arc A257 (-16.4114, 33.4805) -> (-16.2073, 32.5314) centre (0, 36.5125) ccw
  arc A258 (-16.2073, 32.5314) -> (-18.8777, 30.6927) centre (-10.2098, 20.9625) ccw
  arc A259 (-18.8777, 30.6927) -> (-18.5074, 29.6049) centre (0, 36.5125) ccw
  arc A260 (-18.5074, 29.6049) -> (-15.2698, 29.7775) centre (-17.577, 42.6027) ccw
  arc A261 (-15.2698, 29.7775) -> (-14.8523, 28.9011) centre (0, 36.5125) ccw
  arc A262 (-14.8523, 28.9011) -> (-17.0267, 26.4961) centre (-6.3485, 19.0272) ccw
  arc A263 (-17.0267, 26.4961) -> (-16.4155, 25.523) centre (0, 36.5125) ccw
  arc A264 (-16.4155, 25.523) -> (-13.305, 26.4376) centre (-18.5077, 38.385) ccw
  arc A265 (-13.305, 26.4376) -> (-12.6967, 25.681) centre (0, 36.5125) ccw
  arc A266 (-12.6967, 25.681) -> (-14.2578, 22.8394) centre (-2.145, 18.0344) ccw
  arc A267 (-14.2578, 22.8394) -> (-13.4387, 22.0336) centre (0, 36.5125) ccw
  arc A268 (-13.4387, 22.0336) -> (-10.6229, 23.6408) centre (-18.4406, 34.0664) ccw
  arc A269 (-10.6229, 23.6408) -> (-9.8565, 23.045) centre (0, 36.5125) ccw
  arc A270 (-9.8565, 23.045) -> (-10.7203, 19.9199) centre (2.1742, 18.0378) ccw
  arc A271 (-10.7203, 19.9199) -> (-9.7374, 19.3247) centre (0, 36.5125) ccw
  arc A272 (-9.7374, 19.3247) -> (-7.3682, 21.538) centre (-17.3795, 29.8796) ccw
  arc A273 (-7.3682, 21.538) -> (-6.485, 21.1349) centre (0, 36.5125) ccw
  arc A274 (-6.485, 21.1349) -> (-6.6048, 17.8949) centre (6.3761, 19.0372) ccw
  arc A275 (-6.6048, 17.8949) -> (-5.5111, 17.5424) centre (0, 36.5125) ccw
  arc A276 (-5.5111, 17.5424) -> (-3.7162, 20.2424) centre (-15.3813, 26.0504) ccw
  arc A277 (-3.7162, 20.2424) -> (-2.7639, 20.0539) centre (0, 36.5125) ccw
  arc A278 (-2.7639, 20.0539) -> (-2.1332, 16.8736) centre (10.2343, 20.9787) ccw
  arc A279 (-2.1332, 16.8736) -> (-0.9877, 16.7828) centre (0, 36.5125) ccw
  arc A280 (-0.9877, 16.7828) -> (0.1361, 19.824) centre (-12.554, 22.7853) ccw
  arc A281 (0.1361, 19.824) -> (1.1062, 19.8601) centre (0, 36.5125) ccw
  arc A282 (1.1062, 19.8601) -> (2.4533, 16.911) centre (13.5408, 23.7576) ccw
  arc A283 (2.4533, 16.911) -> (3.5889, 17.0868) centre (0, 36.5125) ccw
  arc A284 (3.5889, 17.0868) -> (3.9811, 20.3052) centre (-9.0499, 20.2601) ccw
  arc A285 (3.9811, 20.3052) -> (4.9167, 20.5641) centre (0, 36.5125) ccw
  arc A286 (4.9167, 20.5641) -> (6.9076, 18.0051) centre (16.1173, 27.2242) ccw
  arc A287 (6.9076, 18.0051) -> (7.972, 18.4381) centre (0, 36.5125) ccw
  arc A288 (7.972, 18.4381) -> (7.6114, 21.6602) centre (-5.0579, 18.6112) ccw
  arc A289 (7.6114, 21.6602) -> (8.4622, 22.1279) centre (0, 36.5125) ccw
  arc A290 (8.4622, 22.1279) -> (10.9895, 20.097) centre (17.8249, 31.1914) ccw
  arc A291 (10.9895, 20.097) -> (11.9254, 20.7637) centre (0, 36.5125) ccw
  arc A292 (11.9254, 20.7637) -> (10.8315, 23.8158) centre (-0.7932, 17.9273) ccw
  arc A293 (10.8315, 23.8158) -> (11.5514, 24.4671) centre (0, 36.5125) ccw
  arc A294 (11.5514, 24.4671) -> (14.4789, 23.0738) centre (18.5715, 35.4456) ccw
  arc A295 (14.4789, 23.0738) -> (15.2358, 23.9384) centre (0, 36.5125) ccw
  arc A296 (15.2358, 23.9384) -> (13.4675, 26.656) centre (3.5142, 18.2453) ccw
  arc A297 (13.4675, 26.656) -> (14.0179, 27.4557) centre (0, 36.5125) ccw
  arc A298 (14.0179, 27.4557) -> (17.1878, 26.7751) centre (18.317, 39.7572) ccw
  arc A299 (17.1878, 26.7751) -> (17.7249, 27.791) centre (0, 36.5125) ccw
  arc A300 (17.7249, 27.791) -> (15.3776, 30.0275) centre (7.6322, 19.5481) ccw
  arc A301 (15.3776, 30.0275) -> (15.7287, 30.9326) centre (0, 36.5125) ccw
  arc A302 (15.7287, 30.9326) -> (18.9701, 31.0014) centre (17.075, 43.8939) ccw
  arc A303 (18.9701, 31.0014) -> (19.2585, 32.1137) centre (0, 36.5125) ccw
  arc A304 (19.2585, 32.1137) -> (16.4586, 33.7486) centre (11.3387, 21.7655) ccw
  arc A305 (16.4586, 33.7486) -> (16.5915, 34.7103) centre (0, 36.5125) ccw
  arc A306 (16.5915, 34.7103) -> (19.7297, 35.5248) centre (14.9124, 47.6327) ccw
  arc A307 (19.7297, 35.5248) -> (19.7538, 36.6736) centre (0, 36.5125) ccw
  arc A308 (19.7538, 36.6736) -> (16.6524, 37.6187) centre (14.434, 24.7779) ccw
  arc A309 (16.6524, 37.6187) -> (16.5599, 38.5851) centre (0, 36.5125) ccw
  arc A310 (16.5599, 38.5851) -> (19.4257, 40.1014) centre (11.946, 50.772) ccw
  arc A311 (19.4257, 40.1014) -> (19.1842, 41.2248) centre (0, 36.5125) ccw
  arc A312 (19.1842, 41.2248) -> (15.9484, 41.4292) centre (16.7511, 28.4229) ccw
  arc A313 (15.9484, 41.4292) -> (15.6355, 42.3482) centre (0, 36.5125) ccw
  arc A314 (15.6355, 42.3482) -> (18.0744, 44.4845) centre (8.3355, 53.1426) ccw
  arc A315 (18.0744, 44.4845) -> (17.5803, 45.522) centre (0, 36.5125) ccw
  arc A316 (17.5803, 45.522) -> (14.3846, 44.9747) centre (18.1651, 32.504) ccw
  arc A317 (14.3846, 44.9747) -> (13.8683, 45.7967) centre (0, 36.5125) ccw
  arc A318 (13.8683, 45.7967) -> (15.7488, 48.4379) centre (4.2756, 54.6166) ccw
  arc A319 (15.7488, 48.4379) -> (15.0287, 49.3334) centre (0, 36.5125) ccw
  arc A320 (15.0287, 49.3334) -> (12.0454, 48.0639) centre (18.5999, 36.8012) ccw
  arc A321 (12.0454, 48.0639) -> (11.3534, 48.7447) centre (0, 36.5125) ccw
  arc A322 (11.3534, 48.7447) -> (12.5741, 51.7483) centre (-0.0147, 55.1147) ccw
  arc A323 (12.5741, 51.7483) -> (11.6669, 52.4537) centre (0, 36.5125) ccw
  arc A324 (11.6669, 52.4537) -> (9.0568, 50.5304) centre (18.032, 41.0829) ccw
  arc A325 (9.0568, 50.5304) -> (8.2264, 51.0333) centre (0, 36.5125) ccw
  arc A326 (8.2264, 51.0333) -> (8.7215, 54.2374) centre (-4.3043, 54.6098) ccw
  arc A327 (8.7215, 54.2374) -> (7.6761, 54.7146) centre (0, 36.5125) ccw
  arc A328 (7.6761, 54.7146) -> (5.5799, 52.2412) centre (16.4919, 45.1181) ccw
  arc A329 (5.5799, 52.2412) -> (4.6559, 52.539) centre (0, 36.5125) ccw
  arc A330 (4.6559, 52.539) -> (4.3988, 55.771) centre (-8.3618, 53.1294) ccw
  arc A331 (4.3988, 55.771) -> (3.2715, 55.9942) centre (0, 36.5125) ccw
  arc A332 (3.2715, 55.9942) -> (2.0499, 53.7393) centre (14.0628, 48.6895) ccw
  arc A333 (2.0499, 53.7393) -> (2.0132, 53.6005) centre (21.343, 48.566) ccw
  arc A334 (2.0132, 53.6005) -> (1.9924, 53.6003) centre (2.7056, -36.0971) ccw
  arc A335 (1.9924, 53.6003) -> (1.8022, 53.104) centre (14.0628, 48.6895) ccw
  arc A336 (1.8022, 53.104) -> (0.8345, 53.1807) centre (0, 36.5125) ccw
  arc A337 (0.8345, 53.1807) -> (-0.1611, 56.2663) centre (-11.9685, 50.7531) ccw
  arc A338 (-0.1611, 56.2663) -> (-1.3094, 56.2235) centre (0, 36.5125) ccw
  arc A339 (-1.3094, 56.2235) -> (-2.0726, 53.0724) centre (10.8755, 51.6043) ccw
  arc A340 (-2.0726, 53.0724) -> (-3.032, 52.9239) centre (0, 36.5125) ccw
  arc A341 (-3.032, 52.9239) -> (-3.2586, 53.4046) centre (-14.93, 47.6091) ccw
  arc A342 (-3.2586, 53.4046) -> (-3.2794, 53.4032) centre (2.7056, -36.0971) ccw
  arc A343 (-3.2794, 53.4032) -> (-3.3263, 53.5389) centre (-22.1808, 46.9442) ccw
  circle A344 centre (0, 36.5125) radius 5
  line L0 (38.1, -0.0297) -> (-50.6072, -0.0297)
  circle A345 centre (0, -36.572) radius 5
  line L1 (0, 36.5125) -> (0, 72.8686)
  circle A346 centre (0, 72.8686) radius 5
  line L2 (0, -36.572) -> (0, -73.085)
  circle A347 centre (0, -73.085) radius 5
  point P0 (0, 0)
  dimension "d63" = 10
  dimension "d64" = 10
  dimension "d70" = 10
  dimension "d71" = 36.513
  dimension "d72" = 10
  constraints: 456 point on circle, 233 centre point, 6 end point, 4 coincident, 2 vertical, 1 horizontal, 1 symmetric about line, 1 other
  measures "d63" diameter of A229
  measures "d64" diameter of A344
  measures "d70" diameter of A346
  measures "d71" distance of L2.start L2.end
  measures "d72" diameter of A347
extrude "Extrusion5" cut sketch "Sketch6" against normal blind 5 contours A229 A346 | A229 A346 L1 | L1 A346 A229 | A344 | A345 | A347 picked at (-2.6863, 72.0867)
pattern_circular "Circular Pattern2" count 4 over 360 about axis through (0, -10, 0) along (0, 1, 0) of "Extrusion5"
sketch "Sketch7" plane through (-10, 9.6572, 112.525) normal (0, -1, 0) x (1, 0, 0)
  line L0 (10, -112.525) -> (-46.5685, -55.9565)
  line L1 (10, -112.525) -> (90, -112.525) construction
  line L2 (-41.5685, -50.9565) -> (-51.5685, -50.9565)
  line L3 (-51.5685, -50.9565) -> (-51.5685, -60.9565)
  line L4 (-51.5685, -60.9565) -> (-41.5685, -60.9565)
  line L5 (-41.5685, -60.9565) -> (-41.5685, -50.9565)
  line L6 (-41.5685, -50.9565) -> (-51.5685, -60.9565) construction
  line L7 (-51.5685, -50.9565) -> (-41.5685, -60.9565) construction
  line L8 (10, -112.525) -> (70, -112.525) construction
  dimension "d73" = 80
  dimension "d74" = 135
  dimension "d75" = 10
  dimension "d76" = 10
  constraints: 18 end point, 3 horizontal, 2 midpoint, 2 parallel, 1 equal length, 1 perpendicular
  measures "d73" distance of L0.start L0.end
  measures "d74" angle of L1 L0
  measures "d75" distance of L4.end L3.end
  measures "d76" distance of L3.end L2.end
extrude "Extrusion6" cut sketch "Sketch7" against normal blind 3
pattern_circular "Circular Pattern3" count 4 over 360 about axis through (0, -10, 0) along (0, 1, 0) of "Extrusion6"
sketch "Sketch2" plane through (0, 0, 0) normal (1, 0, 0) x (0, 1, 0)
  line L0 (73.5353, 154.0417) -> (-12.7083, 154.0417)
  line L1 (-12.7083, 154.0417) -> (-12.7083, -160.3341)
  line L2 (-12.7083, -160.3341) -> (73.5353, -160.3341)
  line L3 (73.5353, -160.3341) -> (73.5353, 154.0417)
  point P0 (0, 0)
  constraints: 8 end point, 2 parallel, 1 horizontal, 1 perpendicular
extrude "Extrusion1" cut sketch "Sketch2" along normal blind 183.675
sketch "Sketch8" plane through (0, 0, 0) normal (0, 0, 1) x (1, 0, 0)
  line L0 (-180.975, 66.675) -> (171.45, 66.675)
  line L1 (171.45, 66.675) -> (171.45, -20.6375)
  line L2 (171.45, -20.6375) -> (-180.975, -20.6375)
  line L3 (-180.975, -20.6375) -> (-180.975, 66.675)
  point P0 (0, 0)
  constraints: 8 end point, 2 parallel, 1 horizontal, 1 perpendicular
extrude "Extrusion7" [suppressed]
body "Solid1"
